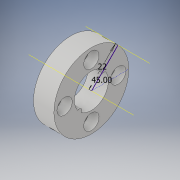
# Autodesk Inventor part: Pen Holder Interface
Saved by Autodesk Inventor 2019 (Build 230136000, 136)
## iProperties
Created: 2019-06-10
Part Number: Pen Holder Interface
Material: Generic
Document SubType Name: Modeling
Designer: Matthew XPS
Density: 1 g/cm^3
Appearance: Default
Author: Matthew XPS
Autodesk Inventor part; units mm, degrees
ref_plane "YZ Plane" through (0, 0, 0) normal (1, 0, 0) x (0, 1, 0)
ref_plane "XZ Plane" through (0, 0, 0) normal (0, 1, 0) x (-1, 0, 0)
ref_plane "XY Plane" through (0, 0, 0) normal (0, 0, 1) x (1, 0, 0)
sketch "Sketch2" plane through (0, 0, 0) normal (1, 0, 0) x (0, 1, 0)
  circle A0 centre (0, 0) radius 10
  circle A1 centre (0, 0) radius 22
  line L0 (0, 0) -> (7.0711, -7.0711)
  line L1 (0, 0) -> (10, 0) construction
  circle A2 centre (7.0711, -7.0711) radius 1.5
  line L2 (0, 0) -> (10.8294, 10.8294)
  line L3 (0, 0) -> (15.315, 0) construction
  circle A3 centre (-7.0711, 7.0711) radius 1.5
  dimension "d3" = 20
  dimension "d4" = 44
  dimension "d16" = 10
  dimension "d17" = 45
  dimension "d18" = 3
  dimension "d19" = 45
  constraints: 8 end point, 4 centre point, 3 coincident, 2 equal length, 2 horizontal, 1 symmetric about line, 1 other
  measures "d3" diameter of A0
  measures "d4" diameter of A1
  measures "d16" distance of L0.start L0.end
  measures "d17" angle of L0 L1
  measures "d18" diameter of A2
  measures "d19" angle of L3 L2
extrude "Extrusion1" add sketch "Sketch2" along normal blind 12 contours A2 A0 | A0 L0 A2 | A3 A0 | A0 A3 | A0 A2 L0 | A1
sketch "Sketch4" plane through (0, 0, 0) normal (1, 0, 0) x (0, 0, -1)
  circle A0 centre (0, 0) radius 15.75
  circle A1 centre (15.75, 0) radius 2.55
  dimension "d9" = 31.5
  dimension "d10" = 5.1
  constraints: 1 centre point, 1 coincident, 1 horizontal alignment, 2 other
  measures "d10" diameter of A1
extrude "Extrusion3" cut sketch "Sketch4" along normal blind 30 contours A0 A1 | A0 A1 picked at (14.9184, -0.4924) picked at (16.4994, -0.6699)
sketch "Sketch5" plane through (12, 0, 0) normal (1, 0, 0) x (0, 0, -1)
  circle A0 centre (15.75, 0) radius 2.55 projected
  circle A1 centre (15.75, 0) radius 4.5
  point P0 (0, 0)
  dimension "d20" = 9
  constraints: 1 centre point, 1 coincident
  measures "d20" diameter of A1
extrude "Extrusion4" cut sketch "Sketch5" against normal blind 6
pattern_circular "Circular Pattern1" count 4 over 360 about axis through (-10, 0, 0) along (1, 0, 0) of "Extrusion3", "Extrusion4"
sketch "Sketch6" plane through (12, 0, 0) normal (1, 0, 0) x (0, 0, -1)
  line L0 (0, 0) -> (15.5563, 15.5563)
  line L1 (0, 0) -> (22, 0) construction
  dimension "d23" = 22
  dimension "d24" = 45
  constraints: 4 end point, 1 equal length, 1 horizontal
  measures "d23" distance of L0.start L0.end
  measures "d24" angle of L1 L0
ref_plane "Work Plane1" through (12, 15.5563, -15.5563) normal (0, 0.7071068, -0.7071068) x (-1, 0, 0)
sketch "Sketch7" plane through (12, 15.5563, -15.5563) normal (0, 0.7071068, -0.7071068) x (-1, 0, 0)
  line L0 (0, 22) -> (0, -22) projected
  line L1 (0, 0) -> (12, 0)
  circle A0 centre (6, 0) radius 2.6
  dimension "d25" = 5.2
  constraints: 2 end point, 2 midpoint, 1 centre point, 1 horizontal
  measures "d25" diameter of A0
extrude "Extrusion5" cut sketch "Sketch7" against normal blind 10
ref_plane "Work Plane2" through (12, 0, 0) normal (0, 0.7071068, -0.7071068) x (-1, 0, 0)
mirror "Mirror1" about plane through (12, 0, 0) normal (0, 0.7071068, -0.7071068) of "Extrusion5"
body "Solid1"
